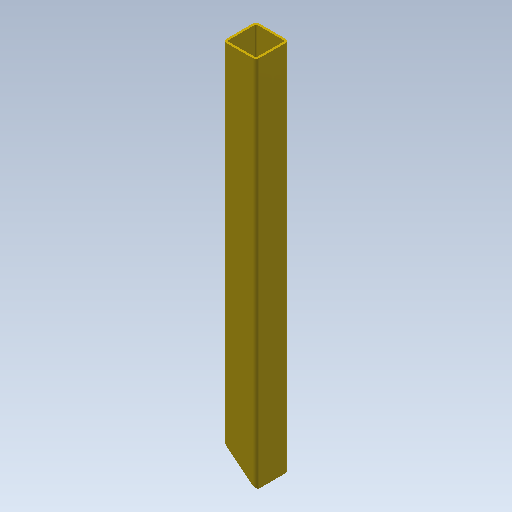
# Autodesk Inventor part: podest duzy profil 5
Saved by Autodesk Inventor 2021 (Build 250183000, 183)
## iProperties
Created: 2024-04-08
Part Number: podest duzy profil 5
Material: Steel
Document SubType Name: Modeling
Designer: Michal
Density: 7.85 g/cm^3
Appearance: Glossy - Gold
Author: Michal
Autodesk Inventor part; units mm, degrees
ref_plane "YZ Plane" through (0, 0, 0) normal (1, 0, 0) x (0, 1, 0)
ref_plane "XZ Plane" through (0, 0, 0) normal (0, 1, 0) x (-1, 0, 0)
sketch "Sketch1" plane through (0, 0, 0) normal (0, 1, 0) x (-1, 0, 0)
  line L0 (-12, 14) -> (12, 14) construction
  line L1 (14, 12) -> (14, -12) construction
  line L2 (12, -14) -> (-12, -14) construction
  line L3 (-14, -12) -> (-14, 12) construction
  line L4 (-14, 14) -> (14, -14) construction
  line L5 (14, 14) -> (-14, -14) construction
  arc A0 (14, 12) -> (12, 14) centre (12, 12) ccw construction
  arc A1 (12, -14) -> (14, -12) centre (12, -12) ccw construction
  arc A2 (-14, -12) -> (-12, -14) centre (-12, -12) ccw construction
  arc A3 (-12, 14) -> (-14, 12) centre (-12, 12) ccw construction
  line L6 (-12, -15) -> (12, -15)
  arc A4 (12, -15) -> (15, -12) centre (12, -12) ccw
  line L7 (15, -12) -> (15, 12)
  arc A5 (15, 12) -> (12, 15) centre (12, 12) ccw
  line L8 (12, 15) -> (-12, 15)
  arc A6 (-12, 15) -> (-15, 12) centre (-12, 12) ccw
  line L9 (-15, 12) -> (-15, -12)
  arc A7 (-15, -12) -> (-12, -15) centre (-12, -12) ccw
  line L10 (13, -12) -> (13, 12)
  arc A8 (13, 12) -> (12, 13) centre (12, 12) ccw
  line L11 (12, 13) -> (-12, 13)
  arc A9 (-12, 13) -> (-13, 12) centre (-12, 12) ccw
  line L12 (-13, 12) -> (-13, -12)
  arc A10 (-13, -12) -> (-12, -13) centre (-12, -12) ccw
  line L13 (-12, -13) -> (12, -13)
  arc A11 (12, -13) -> (13, -12) centre (12, -12) ccw
  point P0 (0, 0)
  point P1 (0, 0)
  point P2 (0, 0)
  dimension "d10" = 2
  dimension "depth" = 30
  dimension "width" = 30
  dimension "thickness" = 2
  constraints: 28 end point, 24 point on circle, 12 centre point, 8 point on line, 8 tangent, 6 parallel, 3 equal radius, 3 midpoint, 3 perpendicular, 1 coincident, 1 horizontal, 15 other
  measures "d10" radius of A0
  measures "depth" distance between parallel lines of L6 L8
  measures "width" distance between parallel lines of L9 L7
  measures "thickness" distance between parallel lines of L10 L7
extrude "Extrusion1" add sketch "Sketch1" along normal blind 1000
ref_plane "Work Plane1" through (0, 500, 0) normal (0, -1, 0) x (1, 0, 0)
sketch "Sketch5" plane through (12, 0, -15) normal (0, 0, -1) x (-1, 0, 0)
  arc A0 (-603, 460) -> (-603, 2430) centre (-603, 1445) ccw projected
  line L0 (27, 0) -> (27, 1000) projected
  line L1 (-3, 0) -> (-3, 1000) projected
  line L2 (0, 0) -> (24, 0) projected
  line L3 (0, 0) -> (-3, 0) projected
  line L4 (27, 0) -> (24, 0) projected
  point P0 (12, 0)
  point P1 (27, 687.8177)
  point P2 (-3, 663.831)
extrude "Extrusion4" cut sketch "Sketch5" against normal through all
equation "\"d10\" = thickness"
body "Solid1"
